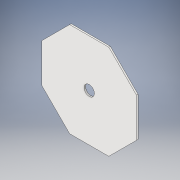
# Autodesk Inventor part: 프레임위밑판
Saved by Autodesk Inventor 2019 (Build 230136000, 136)
## iProperties
Created: 2021-07-09
Part Number: 프레임위밑판
Material: PLA 플라스틱
Document SubType Name: Modeling
Designer: msj19
Density: 1.25 g/cm^3
Appearance: 일반
Author: msj19
Autodesk Inventor part; units mm, degrees
ref_plane "우측면도" through (0, 0, 0) normal (1, 0, 0) x (0, 1, 0)
ref_plane "평면도" through (0, 0, 0) normal (0, 1, 0) x (-1, 0, 0)
ref_plane "정면도" through (0, 0, 0) normal (0, 0, 1) x (1, 0, 0)
sketch "스케치1" plane through (0, 0, 0) normal (0, 0, 1) x (1, 0, 0)
  circle A0 centre (0, 0) radius 98.462
  line L0 (37.6798, 90.967) -> (90.967, 37.6798)
  line L1 (90.967, 37.6798) -> (90.967, -37.6798)
  line L2 (90.967, -37.6798) -> (37.6798, -90.967)
  line L3 (37.6798, -90.967) -> (-37.6798, -90.967)
  line L4 (-37.6798, -90.967) -> (-90.967, -37.6798)
  line L5 (-90.967, -37.6798) -> (-90.967, 37.6798)
  line L6 (-90.967, 37.6798) -> (-37.6798, 90.967)
  line L7 (-37.6798, 90.967) -> (37.6798, 90.967)
  circle A1 centre (0, 0) radius 10
  dimension "d16" = 196.924
  dimension "d17" = 20
  constraints: 16 end point, 3 coincident, 1 centre point, 1 horizontal, 20 other
  measures "d17" diameter of A1
extrude "돌출1" add sketch "스케치1" against normal blind 3 contours L1 L2 L3 L4 L5 L6 L7 L0
